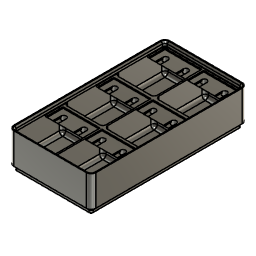
Center 2x3x2 v14 (Autodesk Fusion 360 design; units mm, degrees)
Autodesk Fusion 360 part; units mm, degrees
note: some values were not read from the file. Chosen so that the rebuilt part matches the saved one: that a step has no effect.
ref_plane "Piano di lavoro1" through (0, 0, 0) normal (0, 0, 1) x (1, 0, 0) in component "Gridfinity bin 1x1x3"
sketch "Schizzo1" plane through (0, 0, 0) normal (0, 0, 1) x (1, 0, 0) in component "Gridfinity bin 1x1x3"
  line L0 (-0.25, -0.25) -> (64.75, -0.25)
  line L1 (64.75, -0.25) -> (64.75, 122.75)
  line L2 (64.75, 122.75) -> (-0.25, 122.75)
  line L3 (-0.25, 122.75) -> (-0.25, -0.25)
  dimension "d1438" = 0.25
  dimension "d1439" = 0.25
  dimension "d1440" = 65
  dimension "d1441" = 123
  constraint horizontal L0
  constraint vertical L1
  constraint horizontal L2
  constraint vertical L3
  measures "d1438" vertical distance of origin L0.start
  measures "d1439" horizontal distance of origin L2.end
  measures "d1440" horizontal distance of L0.start L0.end
  measures "d1441" vertical distance of L0.end L1.end
extrude "Base top section extrude" add sketch "Schizzo1" against normal blind 2.4 makes body 1 in component "Gridfinity bin 1x1x3"
fillet "Base corner fillet" radius 4 8 edges at (-0.25, -0.25, -1.2) (64.75, -0.25, -1.2) (64.75, -0.25, -1.2) (64.75, 122.75, -1.2) (64.75, 122.75, -1.2) (-0.25, 122.75, -1.2) (-0.25, 122.75, -1.2) (-0.25, -0.25, -1.2) on bodies 1 in component "Gridfinity bin 1x1x3"
chamfer "Smusso1" distance 2.4 angle 45 8 edges at (0.9216, 121.5784, -2.4) (-0.25, 61.25, -2.4) (0.9216, 0.9216, -2.4) (32.25, -0.25, -2.4) (63.5784, 0.9216, -2.4) (64.75, 61.25, -2.4) (63.5784, 121.5784, -2.4) (32.25, 122.75, -2.4) on bodies 1 in component "Gridfinity bin 1x1x3"
extrude "Estrusione2" add 1 faces at (42.2835, 42.0833, -2.4) along direction (0, 0, -1) blind 2.6 on bodies 1 bodies 1 in component "Gridfinity bin 1x1x3"
chamfer "Smusso2" distance 0.8 angle 45 8 edges at (2.6186, 119.8814, -5) (32.25, 120.35, -5) (61.8814, 119.8814, -5) (62.35, 61.25, -5) (61.8814, 2.6186, -5) (32.25, 2.15, -5) (2.6186, 2.6186, -5) (2.15, 61.25, -5) on bodies 1 in component "Gridfinity bin 1x1x3"
pattern_linear "Serie R1" [no effect] in component "Gridfinity bin 1x1x3"
sketch "Schizzo2" plane through (0, 0, 0) normal (0, 0, 1) x (1, 0, 0) in component "Gridfinity bin 1x1x3"
  line L0 (0, 0) -> (64.5, 0)
  line L1 (64.5, 0) -> (64.5, 122.5)
  line L2 (64.5, 122.5) -> (0, 122.5)
  line L3 (0, 122.5) -> (0, 0)
  dimension "d1454" = 64.5
  dimension "d1455" = 122.5
  constraint horizontal L0
  constraint vertical L1
  constraint horizontal L2
  constraint vertical L3
  constraint coincident L0.start L3
  constraint coincident L3.end L0
  measures "d1454" horizontal distance of L0.start L0.end
  measures "d1455" vertical distance of L0.end L1.end
extrude "Simple box extrude" add sketch "Schizzo2" along normal blind 20.2 separate body makes body 2 in component "Gridfinity bin 1x1x3"
fillet "Bin body corner fillets" radius 3.75 8 edges at (0, 122.5, 10.1) (64.5, 122.5, 10.1) (64.5, 0, 10.1) (0, 0, 10.1) (0, 0, 10.1) (0, 122.5, 10.1) (64.5, 122.5, 10.1) (64.5, 0, 10.1) on bodies 2 in component "Gridfinity bin 1x1x3"
ref_plane "Piano di lavoro2" through (0, 0, 20.2) normal (0, 0, 1) x (1, 0, 0) in component "Gridfinity bin 1x1x3"
sketch "Schizzo3" plane through (0, 0, 20.2) normal (0, 0, 1) x (1, 0, 0) in component "Gridfinity bin 1x1x3"
  line L0 (0, 0) -> (64.5, 0)
  line L1 (64.5, 0) -> (64.5, 122.5)
  line L2 (64.5, 122.5) -> (0, 122.5)
  line L3 (0, 122.5) -> (0, 0)
  dimension "d1461" = 64.5
  dimension "d1462" = 122.5
  constraint horizontal L0
  constraint vertical L1
  constraint horizontal L2
  constraint vertical L3
  constraint coincident L0.start L3
  constraint coincident L3.end L0
  measures "d1461" horizontal distance of L0.start L0.end
  measures "d1462" vertical distance of L0.end L1.end
extrude "Simple box at point extrude" add sketch "Schizzo3" along normal blind 4.4 separate body makes body 3 in component "Gridfinity bin 1x1x3"
fillet "Lip body corner fillets" radius 3.75 8 edges at (0, 122.5, 22.4) (64.5, 122.5, 22.4) (64.5, 122.5, 22.4) (64.5, 0, 22.4) (64.5, 0, 22.4) (0, 0, 22.4) (0, 0, 22.4) (0, 122.5, 22.4) on bodies 3 in component "Gridfinity bin 1x1x3"
ref_plane "Piano di lavoro3" through (0, 0, 25.2) normal (0, 0, 1) x (1, 0, 0) in component "Gridfinity bin 1x1x3"
sketch "Schizzo4" plane through (0, 0, 25.2) normal (0, 0, 1) x (1, 0, 0) in component "Gridfinity bin 1x1x3"
  line L0 (-0.5, -0.5) -> (65, -0.5)
  line L1 (65, -0.5) -> (65, 123)
  line L2 (65, 123) -> (-0.5, 123)
  line L3 (-0.5, 123) -> (-0.5, -0.5)
  dimension "d1468" = 0.5
  dimension "d1469" = 0.5
  dimension "d1470" = 65.5
  dimension "d1471" = 123.5
  constraint horizontal L0
  constraint vertical L1
  constraint horizontal L2
  constraint vertical L3
  measures "d1468" vertical distance of origin L0.start
  measures "d1469" horizontal distance of origin L2.end
  measures "d1470" horizontal distance of L0.start L0.end
  measures "d1471" vertical distance of L0.end L1.end
extrude "Base top section extrude (1)" add sketch "Schizzo4" against normal blind 2.4 separate body makes body 4 in component "Gridfinity bin 1x1x3"
fillet "Base corner fillet (1)" radius 4.25 8 edges at (-0.5, -0.5, 24) (65, -0.5, 24) (65, -0.5, 24) (65, 123, 24) (65, 123, 24) (-0.5, 123, 24) (-0.5, 123, 24) (-0.5, -0.5, 24) on bodies 4 in component "Gridfinity bin 1x1x3"
chamfer "Smusso3" distance 2.4 angle 45 8 edges at (0.7448, 121.7552, 22.8) (-0.5, 61.25, 22.8) (0.7448, 0.7448, 22.8) (32.25, -0.5, 22.8) (63.7552, 0.7448, 22.8) (65, 61.25, 22.8) (63.7552, 121.7552, 22.8) (32.25, 123, 22.8) on bodies 4 in component "Gridfinity bin 1x1x3"
extrude "Estrusione6" add 1 faces at (42.3668, 80.4167, 22.8) along direction (0, 0, -1) blind 2.6 on bodies 4 bodies 4 in component "Gridfinity bin 1x1x3"
ref_plane "Piano di lavoro4" through (32.25, 61.25, 24.6) normal (0, 0, 1) x (1, 0, 0) in component "Gridfinity bin 1x1x3"
sketch "Schizzo5" plane through (0, 0, 24.6) normal (0, 0, 1) x (1, 0, 0) in component "Gridfinity bin 1x1x3"
  line L0 (0, 0) -> (64.5, 0)
  line L1 (64.5, 0) -> (64.5, 122.5)
  line L2 (64.5, 122.5) -> (0, 122.5)
  line L3 (0, 122.5) -> (0, 0)
  dimension "d1480" = 64.5
  dimension "d1481" = 122.5
  constraint horizontal L0
  constraint vertical L1
  constraint horizontal L2
  constraint vertical L3
  constraint coincident L0.start L3
  constraint coincident L3.end L0
  measures "d1480" horizontal distance of L0.start L0.end
  measures "d1481" vertical distance of L0.end L1.end
extrude "Lip top chamfer cut" add sketch "Schizzo5" against normal blind 0.6 separate body makes body 5 in component "Gridfinity bin 1x1x3"
combine "Combina1" operation cut target body 3 tool bodies 5 4 in component "Gridfinity bin 1x1x3"
ref_plane "Piano di lavoro5" through (0, 0, 20.2) normal (0, 0, 1) x (1, 0, 0) in component "Gridfinity bin 1x1x3"
sketch "Schizzo6" plane through (0, 0, 20.2) normal (0, 0, 1) x (1, 0, 0) in component "Gridfinity bin 1x1x3"
  line L0 (1.2, 1.9) -> (63.3, 1.9)
  line L1 (63.3, 1.9) -> (63.3, 121.3)
  line L2 (63.3, 121.3) -> (1.2, 121.3)
  line L3 (1.2, 121.3) -> (1.2, 1.9)
  dimension "d1485" = 1.9
  dimension "d1486" = 1.2
  dimension "d1487" = 62.1
  dimension "d1488" = 119.4
  constraint horizontal L0
  constraint vertical L1
  constraint horizontal L2
  constraint vertical L3
  measures "d1485" vertical distance of origin L0.start
  measures "d1486" horizontal distance of origin L2.end
  measures "d1487" horizontal distance of L0.start L0.end
  measures "d1488" vertical distance of L0.end L1.end
extrude "Lip bottom chamfer extrude" add sketch "Schizzo6" along normal blind 2.55 separate body makes body 6 in component "Gridfinity bin 1x1x3"
fillet "Raccordo5" radius 2.55 8 edges at (1.2, 121.3, 21.475) (63.3, 121.3, 21.475) (1.2, 1.9, 21.475) (1.2, 121.3, 21.475) (63.3, 121.3, 21.475) (63.3, 1.9, 21.475) (63.3, 1.9, 21.475) (1.2, 1.9, 21.475) on bodies 6 in component "Gridfinity bin 1x1x3"
chamfer "Smusso4" distance 2.55 angle 45 5 edges at (63.3, 61.6, 22.75) (62.5531, 120.5531, 22.75) (32.25, 121.3, 22.75) (1.9469, 120.5531, 22.75) (1.2, 61.6, 22.75) on bodies 6 in component "Gridfinity bin 1x1x3"
combine "Combina2" operation cut target body 3 tool bodies 6 in component "Gridfinity bin 1x1x3"
ref_plane "Piano di lavoro6" through (0, 0, 20.2) normal (0, 0, 1) x (1, 0, 0) in component "Gridfinity bin 1x1x3"
sketch "Schizzo7" plane through (0, 0, 20.2) normal (0, 0, 1) x (1, 0, 0) in component "Gridfinity bin 1x1x3"
  line L0 (1.2, 1.9) -> (31.65, 1.9)
  line L1 (31.65, 1.9) -> (31.65, 40.9)
  line L2 (31.65, 40.9) -> (1.2, 40.9)
  line L3 (1.2, 40.9) -> (1.2, 1.9)
  dimension "d1495" = 1.9
  dimension "d1496" = 1.2
  dimension "d1497" = 30.45
  dimension "d1498" = 39
  constraint horizontal L0
  constraint vertical L1
  constraint horizontal L2
  constraint vertical L3
  measures "d1495" vertical distance of origin L0.start
  measures "d1496" horizontal distance of origin L2.end
  measures "d1497" horizontal distance of L0.start L0.end
  measures "d1498" vertical distance of L0.end L1.end
extrude "Inner cutout extrude" add sketch "Schizzo7" against normal blind 19.2 separate body makes body 7 in component "Gridfinity bin 1x1x3"
fillet "Raccordo6" radius 16 1 edges at (16.425, 1.9, 1) on bodies 7 in component "Gridfinity bin 1x1x3"
fillet "Raccordo7" radius 2.55 16 edges at (1.2, 1.9, 18.6) (1.2, 6.5863, 5.6863) (1.2, 29.4, 1) (1.2, 40.9, 10.6) (31.65, 1.9, 18.6) (31.65, 6.5863, 5.6863) (31.65, 29.4, 1) (1.2, 1.9, 18.6) (1.2, 6.5863, 5.6863) (1.2, 29.4, 1) (31.65, 40.9, 10.6) (31.65, 1.9, 18.6) (31.65, 6.5863, 5.6863) (31.65, 29.4, 1) (31.65, 40.9, 10.6) (1.2, 40.9, 10.6) on bodies 7 in component "Gridfinity bin 1x1x3"
fillet "Raccordo8" radius 2.55 3 edges at (16.425, 40.9, 1) (30.9031, 40.1531, 1.7469) (1.9469, 40.1531, 1.7469) on bodies 7 in component "Gridfinity bin 1x1x3"
ref_plane "Piano di lavoro7" through (1.2, 0, 0) normal (1, 0, 0) x (0, 1, 0) in component "Gridfinity bin 1x1x3"
sketch "Schizzo8" plane through (1.2, 0, 0) normal (1, 0, 0) x (0, 0, -1) in component "Gridfinity bin 1x1x3"
  line L0 (-19.7, 40.9) -> (-5.2515, 40.9)
  line L1 (-19.7, 40.9) -> (-19.7, 26.4515)
  line L2 (-5.2515, 40.9) -> (-19.7, 26.4515)
  dimension "d1508" = 40.9
  dimension "d1509" = 19.7
  dimension "d1510" = 14.4485
  dimension "d1511" = 135
  constraint horizontal L0
  constraint vertical L1
  constraint coincident L0.start L1.start
  constraint coincident L1.end L2.end
  constraint coincident L0.end L2.start
  measures "d1508" vertical distance of origin L0.start
  measures "d1509" horizontal distance of origin L0.start
  measures "d1510" vertical distance of L0.start L1.end
  measures "d1511" angle of L0 L2
extrude "Estrusione10" add sketch "Schizzo8" along normal blind 65 separate body makes body 8 in component "Gridfinity bin 1x1x3"
fillet "label tab fillet" radius 0.6 1 edges at (33.7, 26.4515, 19.7) on bodies 8 in component "Gridfinity bin 1x1x3"
combine "Combina3" operation intersect target body 8 tool bodies 7 keep tools in component "Gridfinity bin 1x1x3"
ref_plane "Piano di lavoro8" through (0, 0, 20.2) normal (0, 0, 1) x (1, 0, 0) in component "Gridfinity bin 1x1x3"
sketch "Schizzo9" plane through (0, 0, 20.2) normal (0, 0, 1) x (1, 0, 0) in component "Gridfinity bin 1x1x3"
  line L0 (1.2, 42.1) -> (31.65, 42.1)
  line L1 (31.65, 42.1) -> (31.65, 81.1)
  line L2 (31.65, 81.1) -> (1.2, 81.1)
  line L3 (1.2, 81.1) -> (1.2, 42.1)
  dimension "d1517" = 42.1
  dimension "d1518" = 1.2
  dimension "d1519" = 30.45
  dimension "d1520" = 39
  constraint horizontal L0
  constraint vertical L1
  constraint horizontal L2
  constraint vertical L3
  measures "d1517" vertical distance of origin L0.start
  measures "d1518" horizontal distance of origin L2.end
  measures "d1519" horizontal distance of L0.start L0.end
  measures "d1520" vertical distance of L0.end L1.end
extrude "Inner cutout extrude (1)" add sketch "Schizzo9" against normal blind 19.2 separate body makes body 9 in component "Gridfinity bin 1x1x3"
fillet "Raccordo10" radius 16 1 edges at (16.425, 42.1, 1) on bodies 9 in component "Gridfinity bin 1x1x3"
fillet "Raccordo11" radius 2.55 16 edges at (1.2, 42.1, 18.6) (1.2, 46.7863, 5.6863) (1.2, 69.6, 1) (1.2, 81.1, 10.6) (31.65, 42.1, 18.6) (31.65, 46.7863, 5.6863) (31.65, 69.6, 1) (1.2, 42.1, 18.6) (1.2, 46.7863, 5.6863) (1.2, 69.6, 1) (31.65, 81.1, 10.6) (31.65, 42.1, 18.6) (31.65, 46.7863, 5.6863) (31.65, 69.6, 1) (31.65, 81.1, 10.6) (1.2, 81.1, 10.6) on bodies 9 in component "Gridfinity bin 1x1x3"
fillet "Raccordo12" radius 2.55 3 edges at (16.425, 81.1, 1) (30.9031, 80.3531, 1.7469) (1.9469, 80.3531, 1.7469) on bodies 9 in component "Gridfinity bin 1x1x3"
ref_plane "Piano di lavoro9" through (1.2, 0, 0) normal (1, 0, 0) x (0, 1, 0) in component "Gridfinity bin 1x1x3"
sketch "Schizzo10" plane through (1.2, 0, 0) normal (1, 0, 0) x (0, 0, -1) in component "Gridfinity bin 1x1x3"
  line L0 (-19.7, 81.1) -> (-5.2515, 81.1)
  line L1 (-19.7, 81.1) -> (-19.7, 66.6515)
  line L2 (-5.2515, 81.1) -> (-19.7, 66.6515)
  dimension "d1530" = 81.1
  dimension "d1531" = 19.7
  dimension "d1532" = 14.4485
  dimension "d1533" = 135
  constraint horizontal L0
  constraint vertical L1
  constraint coincident L0.start L1.start
  constraint coincident L1.end L2.end
  constraint coincident L0.end L2.start
  measures "d1530" vertical distance of origin L0.start
  measures "d1531" horizontal distance of origin L0.start
  measures "d1532" vertical distance of L0.start L1.end
  measures "d1533" angle of L0 L2
extrude "Estrusione12" add sketch "Schizzo10" along normal blind 65 separate body makes body 10 in component "Gridfinity bin 1x1x3"
fillet "label tab fillet (1)" radius 0.6 1 edges at (33.7, 66.6515, 19.7) on bodies 10 in component "Gridfinity bin 1x1x3"
combine "Combina4" operation intersect target body 10 tool bodies 9 keep tools in component "Gridfinity bin 1x1x3"
ref_plane "Piano di lavoro10" through (0, 0, 20.2) normal (0, 0, 1) x (1, 0, 0) in component "Gridfinity bin 1x1x3"
sketch "Schizzo11" plane through (0, 0, 20.2) normal (0, 0, 1) x (1, 0, 0) in component "Gridfinity bin 1x1x3"
  line L0 (1.2, 82.3) -> (31.65, 82.3)
  line L1 (31.65, 82.3) -> (31.65, 121.3)
  line L2 (31.65, 121.3) -> (1.2, 121.3)
  line L3 (1.2, 121.3) -> (1.2, 82.3)
  dimension "d1539" = 82.3
  dimension "d1540" = 1.2
  dimension "d1541" = 30.45
  dimension "d1542" = 39
  constraint horizontal L0
  constraint vertical L1
  constraint horizontal L2
  constraint vertical L3
  measures "d1539" vertical distance of origin L0.start
  measures "d1540" horizontal distance of origin L2.end
  measures "d1541" horizontal distance of L0.start L0.end
  measures "d1542" vertical distance of L0.end L1.end
extrude "Inner cutout extrude (2)" add sketch "Schizzo11" against normal blind 19.2 separate body makes body 11 in component "Gridfinity bin 1x1x3"
fillet "Raccordo14" radius 16 1 edges at (16.425, 82.3, 1) on bodies 11 in component "Gridfinity bin 1x1x3"
fillet "Raccordo15" radius 2.55 16 edges at (1.2, 82.3, 18.6) (1.2, 86.9863, 5.6863) (1.2, 109.8, 1) (1.2, 121.3, 10.6) (31.65, 82.3, 18.6) (31.65, 86.9863, 5.6863) (31.65, 109.8, 1) (1.2, 82.3, 18.6) (1.2, 86.9863, 5.6863) (1.2, 109.8, 1) (31.65, 121.3, 10.6) (31.65, 82.3, 18.6) (31.65, 86.9863, 5.6863) (31.65, 109.8, 1) (31.65, 121.3, 10.6) (1.2, 121.3, 10.6) on bodies 11 in component "Gridfinity bin 1x1x3"
fillet "Raccordo16" radius 2.55 3 edges at (16.425, 121.3, 1) (30.9031, 120.5531, 1.7469) (1.9469, 120.5531, 1.7469) on bodies 11 in component "Gridfinity bin 1x1x3"
ref_plane "Piano di lavoro11" through (1.2, 0, 0) normal (1, 0, 0) x (0, 1, 0) in component "Gridfinity bin 1x1x3"
sketch "Schizzo12" plane through (1.2, 0, 0) normal (1, 0, 0) x (0, 0, -1) in component "Gridfinity bin 1x1x3"
  line L0 (-19.7, 121.3) -> (-5.2515, 121.3)
  line L1 (-19.7, 121.3) -> (-19.7, 106.8515)
  line L2 (-5.2515, 121.3) -> (-19.7, 106.8515)
  dimension "d1552" = 121.3
  dimension "d1553" = 19.7
  dimension "d1554" = 14.4485
  dimension "d1555" = 135
  constraint horizontal L0
  constraint vertical L1
  constraint coincident L0.start L1.start
  constraint coincident L1.end L2.end
  constraint coincident L0.end L2.start
  measures "d1552" vertical distance of origin L0.start
  measures "d1553" horizontal distance of origin L0.start
  measures "d1554" vertical distance of L0.start L1.end
  measures "d1555" angle of L0 L2
extrude "Estrusione14" add sketch "Schizzo12" along normal blind 65 separate body makes body 12 in component "Gridfinity bin 1x1x3"
fillet "label tab fillet (2)" radius 0.6 1 edges at (33.7, 106.8515, 19.7) on bodies 12 in component "Gridfinity bin 1x1x3"
combine "Combina5" operation intersect target body 12 tool bodies 11 keep tools in component "Gridfinity bin 1x1x3"
ref_plane "Piano di lavoro12" through (0, 0, 20.2) normal (0, 0, 1) x (1, 0, 0) in component "Gridfinity bin 1x1x3"
sketch "Schizzo13" plane through (0, 0, 20.2) normal (0, 0, 1) x (1, 0, 0) in component "Gridfinity bin 1x1x3"
  line L0 (32.85, 1.9) -> (63.3, 1.9)
  line L1 (63.3, 1.9) -> (63.3, 40.9)
  line L2 (63.3, 40.9) -> (32.85, 40.9)
  line L3 (32.85, 40.9) -> (32.85, 1.9)
  dimension "d1561" = 1.9
  dimension "d1562" = 32.85
  dimension "d1563" = 30.45
  dimension "d1564" = 39
  constraint horizontal L0
  constraint vertical L1
  constraint horizontal L2
  constraint vertical L3
  measures "d1561" vertical distance of origin L0.start
  measures "d1562" horizontal distance of origin L2.end
  measures "d1563" horizontal distance of L0.start L0.end
  measures "d1564" vertical distance of L0.end L1.end
extrude "Inner cutout extrude (3)" add sketch "Schizzo13" against normal blind 19.2 separate body makes body 13 in component "Gridfinity bin 1x1x3"
fillet "Raccordo18" radius 16 1 edges at (48.075, 1.9, 1) on bodies 13 in component "Gridfinity bin 1x1x3"
fillet "Raccordo19" radius 2.55 16 edges at (32.85, 1.9, 18.6) (32.85, 6.5863, 5.6863) (32.85, 29.4, 1) (32.85, 40.9, 10.6) (63.3, 1.9, 18.6) (63.3, 6.5863, 5.6863) (63.3, 29.4, 1) (32.85, 1.9, 18.6) (32.85, 6.5863, 5.6863) (32.85, 29.4, 1) (63.3, 40.9, 10.6) (63.3, 1.9, 18.6) (63.3, 6.5863, 5.6863) (63.3, 29.4, 1) (63.3, 40.9, 10.6) (32.85, 40.9, 10.6) on bodies 13 in component "Gridfinity bin 1x1x3"
fillet "Raccordo20" radius 2.55 3 edges at (48.075, 40.9, 1) (62.5531, 40.1531, 1.7469) (33.5969, 40.1531, 1.7469) on bodies 13 in component "Gridfinity bin 1x1x3"
ref_plane "Piano di lavoro13" through (32.85, 0, 0) normal (1, 0, 0) x (0, 1, 0) in component "Gridfinity bin 1x1x3"
sketch "Schizzo14" plane through (32.85, 0, 0) normal (1, 0, 0) x (0, 0, -1) in component "Gridfinity bin 1x1x3"
  line L0 (-19.7, 40.9) -> (-5.2515, 40.9)
  line L1 (-19.7, 40.9) -> (-19.7, 26.4515)
  line L2 (-5.2515, 40.9) -> (-19.7, 26.4515)
  dimension "d1574" = 40.9
  dimension "d1575" = 19.7
  dimension "d1576" = 14.4485
  dimension "d1577" = 135
  constraint horizontal L0
  constraint vertical L1
  constraint coincident L0.start L1.start
  constraint coincident L1.end L2.end
  constraint coincident L0.end L2.start
  measures "d1574" vertical distance of origin L0.start
  measures "d1575" horizontal distance of origin L0.start
  measures "d1576" vertical distance of L0.start L1.end
  measures "d1577" angle of L0 L2
extrude "Estrusione16" add sketch "Schizzo14" along normal blind 65 separate body makes body 14 in component "Gridfinity bin 1x1x3"
fillet "label tab fillet (3)" radius 0.6 1 edges at (65.35, 26.4515, 19.7) on bodies 14 in component "Gridfinity bin 1x1x3"
combine "Combina6" operation intersect target body 14 tool bodies 13 keep tools in component "Gridfinity bin 1x1x3"
ref_plane "Piano di lavoro14" through (0, 0, 20.2) normal (0, 0, 1) x (1, 0, 0) in component "Gridfinity bin 1x1x3"
sketch "Schizzo15" plane through (0, 0, 20.2) normal (0, 0, 1) x (1, 0, 0) in component "Gridfinity bin 1x1x3"
  line L0 (32.85, 42.1) -> (63.3, 42.1)
  line L1 (63.3, 42.1) -> (63.3, 81.1)
  line L2 (63.3, 81.1) -> (32.85, 81.1)
  line L3 (32.85, 81.1) -> (32.85, 42.1)
  dimension "d1583" = 42.1
  dimension "d1584" = 32.85
  dimension "d1585" = 30.45
  dimension "d1586" = 39
  constraint horizontal L0
  constraint vertical L1
  constraint horizontal L2
  constraint vertical L3
  measures "d1583" vertical distance of origin L0.start
  measures "d1584" horizontal distance of origin L2.end
  measures "d1585" horizontal distance of L0.start L0.end
  measures "d1586" vertical distance of L0.end L1.end
extrude "Inner cutout extrude (4)" add sketch "Schizzo15" against normal blind 19.2 separate body makes body 15 in component "Gridfinity bin 1x1x3"
fillet "Raccordo22" radius 16 1 edges at (48.075, 42.1, 1) on bodies 15 in component "Gridfinity bin 1x1x3"
fillet "Raccordo23" radius 2.55 16 edges at (32.85, 42.1, 18.6) (32.85, 46.7863, 5.6863) (32.85, 69.6, 1) (32.85, 81.1, 10.6) (63.3, 42.1, 18.6) (63.3, 46.7863, 5.6863) (63.3, 69.6, 1) (32.85, 42.1, 18.6) (32.85, 46.7863, 5.6863) (32.85, 69.6, 1) (63.3, 81.1, 10.6) (63.3, 42.1, 18.6) (63.3, 46.7863, 5.6863) (63.3, 69.6, 1) (63.3, 81.1, 10.6) (32.85, 81.1, 10.6) on bodies 15 in component "Gridfinity bin 1x1x3"
fillet "Raccordo24" radius 2.55 3 edges at (48.075, 81.1, 1) (62.5531, 80.3531, 1.7469) (33.5969, 80.3531, 1.7469) on bodies 15 in component "Gridfinity bin 1x1x3"
ref_plane "Piano di lavoro15" through (32.85, 0, 0) normal (1, 0, 0) x (0, 1, 0) in component "Gridfinity bin 1x1x3"
sketch "Schizzo16" plane through (32.85, 0, 0) normal (1, 0, 0) x (0, 0, -1) in component "Gridfinity bin 1x1x3"
  line L0 (-19.7, 81.1) -> (-5.2515, 81.1)
  line L1 (-19.7, 81.1) -> (-19.7, 66.6515)
  line L2 (-5.2515, 81.1) -> (-19.7, 66.6515)
  dimension "d1596" = 81.1
  dimension "d1597" = 19.7
  dimension "d1598" = 14.4485
  dimension "d1599" = 135
  constraint horizontal L0
  constraint vertical L1
  constraint coincident L0.start L1.start
  constraint coincident L1.end L2.end
  constraint coincident L0.end L2.start
  measures "d1596" vertical distance of origin L0.start
  measures "d1597" horizontal distance of origin L0.start
  measures "d1598" vertical distance of L0.start L1.end
  measures "d1599" angle of L0 L2
extrude "Estrusione18" add sketch "Schizzo16" along normal blind 65 separate body makes body 16 in component "Gridfinity bin 1x1x3"
fillet "label tab fillet (4)" radius 0.6 1 edges at (65.35, 66.6515, 19.7) on bodies 16 in component "Gridfinity bin 1x1x3"
combine "Combina7" operation intersect target body 16 tool bodies 15 keep tools in component "Gridfinity bin 1x1x3"
ref_plane "Piano di lavoro16" through (0, 0, 20.2) normal (0, 0, 1) x (1, 0, 0) in component "Gridfinity bin 1x1x3"
sketch "Schizzo17" plane through (0, 0, 20.2) normal (0, 0, 1) x (1, 0, 0) in component "Gridfinity bin 1x1x3"
  line L0 (32.85, 82.3) -> (63.3, 82.3)
  line L1 (63.3, 82.3) -> (63.3, 121.3)
  line L2 (63.3, 121.3) -> (32.85, 121.3)
  line L3 (32.85, 121.3) -> (32.85, 82.3)
  dimension "d1605" = 82.3
  dimension "d1606" = 32.85
  dimension "d1607" = 30.45
  dimension "d1608" = 39
  constraint horizontal L0
  constraint vertical L1
  constraint horizontal L2
  constraint vertical L3
  measures "d1605" vertical distance of origin L0.start
  measures "d1606" horizontal distance of origin L2.end
  measures "d1607" horizontal distance of L0.start L0.end
  measures "d1608" vertical distance of L0.end L1.end
extrude "Inner cutout extrude (5)" add sketch "Schizzo17" against normal blind 19.2 separate body makes body 17 in component "Gridfinity bin 1x1x3"
fillet "Raccordo26" radius 16 1 edges at (48.075, 82.3, 1) on bodies 17 in component "Gridfinity bin 1x1x3"
fillet "Raccordo27" radius 2.55 16 edges at (32.85, 82.3, 18.6) (32.85, 86.9863, 5.6863) (32.85, 109.8, 1) (32.85, 121.3, 10.6) (63.3, 82.3, 18.6) (63.3, 86.9863, 5.6863) (63.3, 109.8, 1) (32.85, 82.3, 18.6) (32.85, 86.9863, 5.6863) (32.85, 109.8, 1) (63.3, 121.3, 10.6) (63.3, 82.3, 18.6) (63.3, 86.9863, 5.6863) (63.3, 109.8, 1) (63.3, 121.3, 10.6) (32.85, 121.3, 10.6) on bodies 17 in component "Gridfinity bin 1x1x3"
fillet "Raccordo28" radius 2.55 3 edges at (48.075, 121.3, 1) (62.5531, 120.5531, 1.7469) (33.5969, 120.5531, 1.7469) on bodies 17 in component "Gridfinity bin 1x1x3"
ref_plane "Piano di lavoro17" through (32.85, 0, 0) normal (1, 0, 0) x (0, 1, 0) in component "Gridfinity bin 1x1x3"
sketch "Schizzo18" plane through (32.85, 0, 0) normal (1, 0, 0) x (0, 0, -1) in component "Gridfinity bin 1x1x3"
  line L0 (-19.7, 121.3) -> (-5.2515, 121.3)
  line L1 (-19.7, 121.3) -> (-19.7, 106.8515)
  line L2 (-5.2515, 121.3) -> (-19.7, 106.8515)
  dimension "d1618" = 121.3
  dimension "d1619" = 19.7
  dimension "d1620" = 14.4485
  dimension "d1621" = 135
  constraint horizontal L0
  constraint vertical L1
  constraint coincident L0.start L1.start
  constraint coincident L1.end L2.end
  constraint coincident L0.end L2.start
  measures "d1618" vertical distance of origin L0.start
  measures "d1619" horizontal distance of origin L0.start
  measures "d1620" vertical distance of L0.start L1.end
  measures "d1621" angle of L0 L2
extrude "Estrusione20" add sketch "Schizzo18" along normal blind 65 separate body makes body 18 in component "Gridfinity bin 1x1x3"
fillet "label tab fillet (5)" radius 0.6 1 edges at (65.35, 106.8515, 19.7) on bodies 18 in component "Gridfinity bin 1x1x3"
combine "Combina8" operation intersect target body 18 tool bodies 17 keep tools in component "Gridfinity bin 1x1x3"
ref_plane "Piano di lavoro18" through (0, 0, 20.2) normal (0, 0, 1) x (1, 0, 0) in component "Gridfinity bin 1x1x3"
sketch "Schizzo19" plane through (0, 0, 20.2) normal (0, 0, 1) x (1, 0, 0) in component "Gridfinity bin 1x1x3"
  line L0 (1.2, 1.9) -> (63.3, 1.9)
  line L1 (63.3, 1.9) -> (63.3, 121.3)
  line L2 (63.3, 121.3) -> (1.2, 121.3)
  line L3 (1.2, 121.3) -> (1.2, 1.9)
  dimension "d1627" = 1.9
  dimension "d1628" = 1.2
  dimension "d1629" = 62.1
  dimension "d1630" = 119.4
  constraint horizontal L0
  constraint vertical L1
  constraint horizontal L2
  constraint vertical L3
  measures "d1627" vertical distance of origin L0.start
  measures "d1628" horizontal distance of origin L2.end
  measures "d1629" horizontal distance of L0.start L0.end
  measures "d1630" vertical distance of L0.end L1.end
extrude "Inner cutout extrude (6)" add sketch "Schizzo19" against normal blind 0.5 separate body makes body 19 in component "Gridfinity bin 1x1x3"
fillet "Raccordo30" radius 2.55 8 edges at (1.2, 1.9, 19.95) (63.3, 1.9, 19.95) (63.3, 1.9, 19.95) (63.3, 121.3, 19.95) (63.3, 121.3, 19.95) (1.2, 121.3, 19.95) (1.2, 121.3, 19.95) (1.2, 1.9, 19.95) on bodies 19 in component "Gridfinity bin 1x1x3"
combine "Combina9" operation cut target body 2 tool bodies 7 9 11 13 15 17 19 in component "Gridfinity bin 1x1x3"
combine "Combina10" operation add target body 2 tool bodies 3 8 10 12 14 16 18 in component "Gridfinity bin 1x1x3"
ref_plane "Piano di lavoro19" through (0, 0, 0) normal (0, 0, 1) x (1, 0, 0) in component "Gridfinity bin 1x1x3"
sketch "Schizzo20" plane through (0, 0, 0) normal (0, 0, 1) x (1, 0, 0) in component "Gridfinity bin 1x1x3"
  line L0 (3.75, 0) -> (60.75, 0)
  line L1 (64.5, 3.75) -> (64.5, 118.75)
  line L2 (60.75, 122.5) -> (3.75, 122.5)
  line L3 (0, 118.75) -> (0, 3.75)
  arc A0 (60.75, 0) -> (64.5, 3.75) centre (60.75, 3.75) ccw
  arc A1 (64.5, 118.75) -> (60.75, 122.5) centre (60.75, 118.75) ccw
  arc A2 (3.75, 122.5) -> (0, 118.75) centre (3.75, 118.75) ccw
  arc A3 (0, 3.75) -> (3.75, 0) centre (3.75, 3.75) ccw
  arc A4 (60.75, -10) -> (74.5, 3.75) centre (60.75, 3.75) ccw
  line L4 (74.5, 3.75) -> (74.5, 118.75)
  arc A5 (74.5, 118.75) -> (60.75, 132.5) centre (60.75, 118.75) ccw
  line L5 (60.75, 132.5) -> (3.75, 132.5)
  arc A6 (3.75, 132.5) -> (-10, 118.75) centre (3.75, 118.75) ccw
  line L6 (-10, 118.75) -> (-10, 3.75)
  arc A7 (-10, 3.75) -> (3.75, -10) centre (3.75, 3.75) ccw
  line L7 (3.75, -10) -> (60.75, -10)
  point P0 (64.5, 0)
  point P1 (64.5, 122.5)
  dimension "d1636" = 64.5
  dimension "d1637" = 122.5
  dimension "d1638" = 3.75
  dimension "d1639" = 10
  constraint horizontal L0
  constraint vertical L1
  constraint horizontal L2
  constraint vertical L3
  constraint coincident origin L3
  constraint coincident origin L0
  constraint coincident P0 L0
  constraint coincident P0 L1
  constraint tangent L0 A0
  constraint tangent L1 A0
  constraint coincident P1 L1
  constraint coincident P1 L2
  constraint tangent L1 A1
  constraint tangent L2 A1
  constraint tangent L2 A2
  constraint tangent L3 A2
  constraint tangent L3 A3
  constraint tangent L0 A3
  constraint equal A0 A1
  constraint equal A1 A2
  constraint equal A2 A3
  measures "d1636" horizontal distance of origin P0
  measures "d1637" vertical distance of P0 P1
  measures "d1638" radius of A0
extrude "Base side clearance cut" cut sketch "Schizzo20" along normal blind 1000 and the other way blind 1000 bodies 1 2 in component "Gridfinity bin 1x1x3"
combine "Combina11" operation add target body 2 tool bodies 1 1 in component "Gridfinity bin 1x1x3"
sketch "Schizzo21" plane through (0, 0, 24) normal (0, 0, 1) x (-1, 0, 0) in component "Gridfinity bin 1x1x3"
  arc A0 (-3.75, -121.8) -> (-0.7, -118.75) centre (-3.75, -118.75) ccw
  line L0 (-3.75, -121.8) -> (-60.75, -121.8)
  arc A1 (-63.8, -118.75) -> (-60.75, -121.8) centre (-60.75, -118.75) ccw
  line L1 (-63.8, -118.75) -> (-63.8, -3.75)
  arc A2 (-60.75, -0.7) -> (-63.8, -3.75) centre (-60.75, -3.75) ccw
  line L2 (-60.75, -0.7) -> (-3.75, -0.7)
  arc A3 (-0.7, -3.75) -> (-3.75, -0.7) centre (-3.75, -3.75) ccw
  line L3 (-0.7, -3.75) -> (-0.7, -118.75)
  arc A4 (-64.5, -118.75) -> (-60.75, -122.5) centre (-60.75, -118.75) ccw
  line L4 (-60.75, -122.5) -> (-3.75, -122.5)
  arc A5 (-3.75, -122.5) -> (0, -118.75) centre (-3.75, -118.75) ccw
  line L5 (0, -118.75) -> (0, -3.75)
  arc A6 (0, -3.75) -> (-3.75, 0) centre (-3.75, -3.75) ccw
  line L6 (-3.75, 0) -> (-60.75, 0)
  arc A7 (-60.75, 0) -> (-64.5, -3.75) centre (-60.75, -3.75) ccw
  line L7 (-64.5, -3.75) -> (-64.5, -118.75)
  line L8 (0, -122.5) -> (-64.5, -122.5) construction
  line L9 (-64.5, -122.5) -> (-64.5, 0) construction
  line L10 (-64.5, 0) -> (0, 0) construction
  line L11 (0, 0) -> (0, -122.5) construction
  line L12 (-32.25, -122.5) -> (-32.25, 0) construction
  line L13 (-2.5, -120) -> (-31.5, -120)
  line L14 (-31.5, -120) -> (-31.5, -108)
  line L15 (-31.5, -108) -> (-2.5, -108)
  line L16 (-2.5, -108) -> (-2.5, -120)
  line L17 (-2.5, -108) -> (-31.5, -108)
  line L18 (-31.5, -108) -> (-31.5, -106)
  line L19 (-31.5, -106) -> (-2.5, -106)
  line L20 (-2.5, -106) -> (-2.5, -108)
  line L21 (-2.5, -114) -> (-31.5, -114) construction
  line L22 (-17, -120) -> (-17, -108) construction
  circle A8 centre (-9, -114) radius 2
  circle A9 centre (-25, -114) radius 2
  circle A10 centre (-9, -74) radius 2
  circle A11 centre (-25, -74) radius 2
  line L23 (-2.5, -80) -> (-31.5, -80)
  line L24 (-2.5, -68) -> (-2.5, -80)
  line L25 (-2.5, -68) -> (-31.5, -68)
  line L26 (-31.5, -66) -> (-2.5, -66)
  line L27 (-31.5, -80) -> (-31.5, -68)
  line L28 (-31.5, -68) -> (-31.5, -66)
  line L29 (-2.5, -66) -> (-2.5, -68)
  circle A12 centre (-9, -34) radius 2
  circle A13 centre (-25, -34) radius 2
  line L30 (-2.5, -40) -> (-31.5, -40)
  line L31 (-2.5, -28) -> (-2.5, -40)
  line L32 (-2.5, -28) -> (-31.5, -28)
  line L33 (-31.5, -26) -> (-2.5, -26)
  line L34 (-31.5, -40) -> (-31.5, -28)
  line L35 (-31.5, -28) -> (-31.5, -26)
  line L36 (-2.5, -26) -> (-2.5, -28)
  circle A14 centre (-39.5, -114) radius 2
  circle A15 centre (-55.5, -114) radius 2
  line L37 (-33, -120) -> (-62, -120)
  line L38 (-33, -108) -> (-33, -120)
  line L39 (-33, -108) -> (-62, -108)
  line L40 (-62, -106) -> (-33, -106)
  line L41 (-62, -120) -> (-62, -108)
  line L42 (-62, -108) -> (-62, -106)
  line L43 (-33, -106) -> (-33, -108)
  circle A16 centre (-39.5, -74) radius 2
  circle A17 centre (-55.5, -74) radius 2
  line L44 (-33, -80) -> (-62, -80)
  line L45 (-33, -68) -> (-33, -80)
  line L46 (-33, -68) -> (-62, -68)
  line L47 (-62, -66) -> (-33, -66)
  line L48 (-62, -80) -> (-62, -68)
  line L49 (-62, -68) -> (-62, -66)
  line L50 (-33, -66) -> (-33, -68)
  circle A18 centre (-39.5, -34) radius 2
  circle A19 centre (-55.5, -34) radius 2
  line L51 (-33, -40) -> (-62, -40)
  line L52 (-33, -28) -> (-33, -40)
  line L53 (-33, -28) -> (-62, -28)
  line L54 (-62, -26) -> (-33, -26)
  line L55 (-62, -40) -> (-62, -28)
  line L56 (-62, -28) -> (-62, -26)
  line L57 (-33, -26) -> (-33, -28)
  line L58 (-7, -114) -> (-11, -114)
  line L59 (-11, -114) -> (-11, -106)
  line L60 (-11, -106) -> (-7, -106)
  line L61 (-7, -106) -> (-7, -114)
  line L62 (-27, -114) -> (-23, -114)
  line L63 (-23, -114) -> (-23, -106)
  line L64 (-27, -106) -> (-27, -114)
  line L65 (-23, -106) -> (-27, -106)
  line L66 (-11, -74) -> (-11, -66)
  line L67 (-7, -66) -> (-7, -74)
  line L68 (-7, -74) -> (-11, -74)
  line L69 (-11, -66) -> (-7, -66)
  line L70 (-23, -66) -> (-27, -66)
  line L71 (-23, -74) -> (-23, -66)
  line L72 (-27, -66) -> (-27, -74)
  line L73 (-27, -74) -> (-23, -74)
  line L74 (-11, -34) -> (-11, -26)
  line L75 (-7, -26) -> (-7, -34)
  line L76 (-7, -34) -> (-11, -34)
  line L77 (-11, -26) -> (-7, -26)
  line L78 (-23, -26) -> (-27, -26)
  line L79 (-23, -34) -> (-23, -26)
  line L80 (-27, -26) -> (-27, -34)
  line L81 (-27, -34) -> (-23, -34)
  line L82 (-41.5, -114) -> (-41.5, -106)
  line L83 (-37.5, -106) -> (-37.5, -114)
  line L84 (-37.5, -114) -> (-41.5, -114)
  line L85 (-41.5, -106) -> (-37.5, -106)
  line L86 (-53.5, -106) -> (-57.5, -106)
  line L87 (-53.5, -114) -> (-53.5, -106)
  line L88 (-57.5, -106) -> (-57.5, -114)
  line L89 (-57.5, -114) -> (-53.5, -114)
  line L90 (-41.5, -74) -> (-41.5, -66)
  line L91 (-37.5, -66) -> (-37.5, -74)
  line L92 (-37.5, -74) -> (-41.5, -74)
  line L93 (-41.5, -66) -> (-37.5, -66)
  line L94 (-53.5, -66) -> (-57.5, -66)
  line L95 (-53.5, -74) -> (-53.5, -66)
  line L96 (-57.5, -66) -> (-57.5, -74)
  line L97 (-57.5, -74) -> (-53.5, -74)
  line L98 (-41.5, -34) -> (-41.5, -26)
  line L99 (-37.5, -26) -> (-37.5, -34)
  line L100 (-37.5, -34) -> (-41.5, -34)
  line L101 (-41.5, -26) -> (-37.5, -26)
  line L102 (-53.5, -26) -> (-57.5, -26)
  line L103 (-53.5, -34) -> (-53.5, -26)
  line L104 (-57.5, -26) -> (-57.5, -34)
  line L105 (-57.5, -34) -> (-53.5, -34)
  dimension "d1644" = 2.5
  dimension "d1645" = 0.75
  dimension "d1646" = 2.5
  dimension "d1647" = 12
  dimension "d1648" = 2
  dimension "d1649" = 29
  dimension "d1650" = 4
  dimension "d1651" = 16
  dimension "d1654" = 40
  dimension "d1655" = 30.5
  constraint horizontal L8
  constraint vertical L9
  constraint horizontal L10
  constraint vertical L11
  constraint collinear L5 L11
  constraint collinear L7 L9
  constraint collinear L4 L8
  constraint collinear L6 L10
  constraint midpoint L8 L12.start
  constraint midpoint L10 L12.end
  constraint horizontal L13
  constraint vertical L14
  constraint horizontal L15
  constraint vertical L16
  constraint horizontal L17
  constraint vertical L18
  constraint horizontal L19
  constraint vertical L20
  constraint midpoint L16 L21.start
  constraint midpoint L14 L21.end
  constraint midpoint L13 L22.start
  constraint midpoint L15 L22.end
  constraint coincident L21 A8.centre
  constraint symmetric L22 A8 A9
  constraint collinear L14 L18
  constraint horizontal L58
  constraint vertical L59
  constraint horizontal L60
  constraint vertical L61
  constraint coincident L19 L59.end
  constraint tangent A8 L59
  constraint symmetric L22 L58.start L62.start
  constraint symmetric L22 L58.end L62.end
  constraint symmetric L22 L59.end L63.end
  constraint symmetric L22 L60.end L64.start
  constraint collinear L21 L58
  measures "d1644" distance of L11 L16
  measures "d1645" distance of L12 L14
  measures "d1646" distance of L8 L13
  measures "d1647" distance of L13 L15
  measures "d1648" distance of L15 L19
  measures "d1649" distance of L14 L16
  measures "d1650" diameter of A8
  measures "d1651" distance of A8.centre A9.centre
extrude "Estrusione23" cut sketch "Schizzo21" against normal blind 1 from surface at -4.3 contours L13 L14 L15 L16 L17 A8 A9 L59 L61 L63 L64 | L15 L17 L19 L20 L61 | L15 L17 L18 L19 L64 | L15 L17 A8 L59 L61 | L15 L17 L19 L59 L60 L61 | L15 L17 L19 L63 L64 L65 | L15 L17 A9 L63 L64 | L15 L17 L19 L59 L63 | A10 A11 L23 L24 L25 L27 L66 L67 L71 L72 | A10 L25 L66 L67 | L25 L26 L29 L67 | L25 L26 L66 L67 L69 | L25 L26 L66 L71 | A11 L25 L71 L72 | L25 L26 L70 L71 L72 | L25 L26 L28 L72 | A12 A13 L30 L31 L32 L34 L74 L75 L79 L80 | A12 L32 L74 L75 | L32 L33 L36 L75 | L32 L33 L74 L75 L77 | L32 L33 L74 L79 | A13 L32 L79 L80 | L32 L33 L78 L79 L80 | L32 L33 L35 L80 | A14 A15 L37 L38 L39 L41 L82 L83 L87 L88 | A14 L39 L82 L83 | L39 L40 L43 L83 | L39 L40 L82 L83 L85 | L39 L40 L82 L87 | A15 L39 L87 L88 | L39 L40 L86 L87 L88 | L39 L40 L42 L88 | A16 A17 L44 L45 L46 L48 L90 L91 L95 L96 | A16 L46 L90 L91 | L46 L47 L50 L91 | L46 L47 L90 L91 L93 | L46 L47 L90 L95 | A17 L46 L95 L96 | L46 L47 L94 L95 L96 | L46 L47 L49 L96 | A18 A19 L51 L52 L53 L55 L98 L99 L103 L104 | A18 L53 L98 L99 | L53 L54 L57 L99 | L53 L54 L98 L99 L101 | L53 L54 L98 L103 | A19 L53 L103 L104 | L53 L54 L102 L103 L104 | L53 L54 L56 L104 bodies 2 in component "Gridfinity bin 1x1x3"
extrude "Estrusione24" cut sketch "Schizzo21" against normal blind 15 contours A8 L58 | A8 L58 | A9 L62 | A9 L62 | A10 L68 | A10 L68 | A11 L73 | A11 L73 | A12 L76 | A12 L76 | A13 L81 | A13 L81 | A14 L84 | A14 L84 | A15 L89 | A15 L89 | A16 L92 | A16 L92 | A17 L97 | A17 L97 | A18 L100 | A18 L100 | A19 L105 | A19 L105 bodies 2 in component "Gridfinity bin 1x1x3"
extrude "Estrusione25" cut sketch "Schizzo21" against normal blind 2 from surface at -4.3 contours L15 L17 A8 L59 L61 | L15 L17 L19 L59 L60 L61 | L15 L17 L19 L63 L64 L65 | L15 L17 A9 L63 L64 | A10 L25 L66 L67 | L25 L26 L66 L67 L69 | A11 L25 L71 L72 | L25 L26 L70 L71 L72 | A12 L32 L74 L75 | L32 L33 L74 L75 L77 | A13 L32 L79 L80 | L32 L33 L78 L79 L80 | A14 L39 L82 L83 | L39 L40 L82 L83 L85 | A15 L39 L87 L88 | L39 L40 L86 L87 L88 | A16 L46 L90 L91 | L46 L47 L90 L91 L93 | A17 L46 L95 L96 | L46 L47 L94 L95 L96 | A18 L53 L98 L99 | L53 L54 L98 L99 L101 | A19 L53 L103 L104 | L53 L54 L102 L103 L104 bodies 2 in component "Gridfinity bin 1x1x3"
component "Gridfinity bin 1x1x3" placed x (1, 0, 0) y (0, 1, 0) z (0, 0, 1) at (0, 0, 0)
equation "d1442 = -( 2.40 mm )"
equation "d1472 = -( 2.40 mm )"
equation "d1482 = -( 0.60 mm )"
equation "d1499 = -( 19.20 mm )"
equation "d1521 = -( 19.20 mm )"
equation "d1543 = -( 19.20 mm )"
equation "d1565 = -( 19.20 mm )"
equation "d1587 = -( 19.20 mm )"
equation "d1609 = -( 19.20 mm )"
equation "d1631 = -( 0.50 mm )"
equation "d1646 = d1644"
named bodies: "Base", "Gridfinity bin 1x1x3", "Lip body", "Lip cutout", "Inner cutout", "label tab", "Inner cutout (1)", "label tab (1)", "Inner cutout (2)", "label tab (2)", "Inner cutout (3)", "label tab (3)", "Inner cutout (4)", "label tab (4)", "Inner cutout (5)", "label tab (5)", "Inner cutout (6)"
